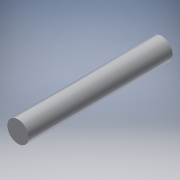
# Autodesk Inventor part: Connecting Rod
Saved by Autodesk Inventor 2016 (Build 200138000, 138)
## iProperties
Created: 2014-03-04
Part Number: Connecting Rod
Material: Aluminum 6061
Document SubType Name: Modeling
Designer: John
Density: 2.71 g/cm^3
Appearance: Aluminum - Flat
Mass: 3.68969 g
Surface Area: 9.20983 cm^2
Volume: 1.36151 cm^3
Author: John
Autodesk Inventor part; units mm, degrees
ref_plane "YZ Plane" through (0, 0, 0) normal (1, 0, 0) x (0, 1, 0)
ref_plane "XZ Plane" through (0, 0, 0) normal (0, 1, 0) x (-1, 0, 0)
ref_plane "XY Plane" through (0, 0, 0) normal (0, 0, 1) x (1, 0, 0)
sketch "Sketch1" plane through (0, 0, 0) normal (0, 0, 1) x (1, 0, 0)
  circle A0 centre (0, 0) radius 3.175
  dimension "d0" = 6.35
  constraints: 1 centre point, 1 coincident
  measures "d0" diameter of A0
extrude "Extrusion1" add sketch "Sketch1" along normal blind 42.9916
body "Solid1"
